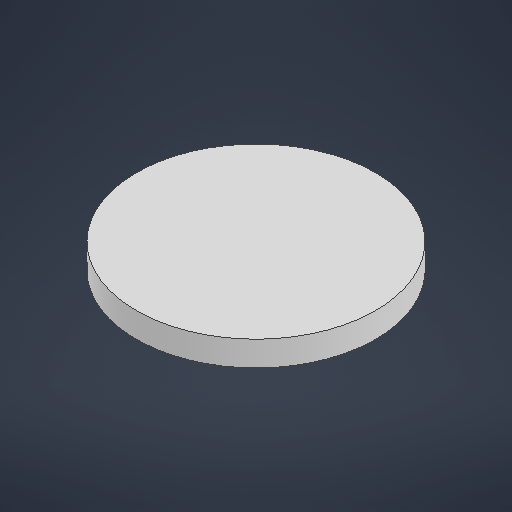
# Autodesk Inventor part: Concave_3_516_Plate
Saved by Autodesk Inventor 2026.1 (Build 301233000, 233)
## iProperties
Created: 2025-12-15
Part Number: Concave_3_516_Plate
Material: Generic
Document SubType Name: Modeling
Designer: usman
Density: 1 g/cm^3
Appearance: Default
Author: usman
Autodesk Inventor part; units mm, degrees
ref_plane "YZ Plane" through (0, 0, 0) normal (1, 0, 0) x (0, 1, 0)
ref_plane "XZ Plane" through (0, 0, 0) normal (0, 1, 0) x (-1, 0, 0)
ref_plane "XY Plane" through (0, 0, 0) normal (0, 0, 1) x (1, 0, 0)
sketch "Sketch1" plane through (0, 0, 0) normal (1, 0, 0) x (0, 1, 0)
  line L0 (6.0547, 0) -> (6.0547, -38.1)
  line L1 (6.0547, -38.1) -> (-1.8828, -38.1)
  line L2 (-1.8828, -38.1) -> (-1.8828, -35.56)
  line L3 (6.0547, 0) -> (-1.0573, 0)
  line L4 (-1.0573, 0) -> (-1.8828, -35.56)
  line L5 (18.8787, 0) -> (-18.455, 0)
  point P0 (0, 0)
  dimension "d0" = 38.1
  dimension "d1" = 7.9375
  dimension "d2" = 2.54
  dimension "d3" = 7.112
  constraints: 12 end point, 3 coincident, 2 horizontal, 2 vertical
  measures "d0" distance of L0.start L0.end
  measures "d1" distance of L0.end L1.end
  measures "d2" distance of L1.end L2.end
  measures "d3" distance of L0.start L3.end
revolve "Revolution1" add sketch "Sketch1" angle 360 about axis through (0, 18.8787, 0) along (0, -1, 0)
body "Solid1"
